Autodesk Inventor part; units mm, degrees
(part 3 of 3)
  spline S565 degree 2 poles (0.1635, 59.9365) (0.1635, 59.319) (1.0898, 58.6191) (1.9646, 58.6191) knots 0 0 0 1 2 2 2
  spline S566 degree 2 poles (1.9646, 58.6191) (2.8085, 58.6191) (3.6987, 59.1543) (3.6987, 59.7461) knots 0 0 0 1 2 2 2
  spline S567 degree 2 poles (3.6987, 59.7461) (3.6987, 60.06) (3.4106, 60.6981) (3.1687, 60.9811) knots 0 0 0 1 2 2 2
  line L445 (4.3265, 63.765) -> (4.3265, 62.9623)
  line L446 (4.3265, 62.9623) -> (-2.3065, 62.9623)
  line L447 (-2.3065, 62.9623) -> (-2.3065, 63.765)
  line L448 (-2.3065, 63.765) -> (4.3265, 63.765)
  spline S568 degree 2 poles (4.4346, 67.0121) (4.4346, 65.8697) (3.1533, 64.6141) (1.9697, 64.6141) knots 0 0 0 1 2 2 2
  spline S569 degree 2 poles (1.9697, 64.6141) (0.8068, 64.6141) (-0.5723, 65.8336) (-0.5723, 66.8165) knots 0 0 0 1 2 2 2
  spline S570 degree 2 poles (-0.5723, 66.8165) (-0.5723, 67.2591) (-0.315, 67.9435) (-0.0423, 68.1956) knots 0 0 0 1 2 2 2
  spline S571 degree 2 poles (-0.0423, 68.1956) (0.2304, 68.4529) (1.0177, 68.7256) (1.5889, 68.7256) knots 0 0 0 1 2 2 2
  line L449 (1.5889, 68.7256) -> (2.0263, 68.7256)
  line L450 (2.0263, 68.7256) -> (2.0263, 65.4271)
  spline S572 degree 2 poles (2.0263, 65.4271) (2.8548, 65.4271) (3.7348, 66.2608) (3.7348, 67.0018) knots 0 0 0 1 2 2 2
  spline S573 degree 2 poles (3.7348, 67.0018) (3.7348, 67.2642) (3.6164, 67.7736) (3.5238, 67.9795) knots 0 0 0 1 2 2 2
  spline S574 degree 2 poles (3.5238, 67.9795) (3.4209, 68.1956) (3.2408, 68.4941) (3.1584, 68.5918) knots 0 0 0 1 2 2 2
  line L451 (3.1584, 68.5918) -> (3.1584, 68.6381)
  line L452 (3.1584, 68.6381) -> (4.0332, 68.6381)
  spline S575 degree 2 poles (4.0332, 68.6381) (4.0898, 68.4992) (4.2545, 68.0772) (4.3008, 67.9126) knots 0 0 0 1 2 2 2
  spline S576 degree 2 poles (4.3008, 67.9126) (4.3677, 67.681) (4.4346, 67.3002) (4.4346, 67.0121) knots 0 0 0 1 2 2 2
  spline S577 degree 2 poles (1.414, 67.9435) (1.0898, 67.9332) (0.6164, 67.7994) (0.4568, 67.6707) knots 0 0 0 1 2 2 2
  spline S578 degree 2 poles (0.4568, 67.6707) (0.2767, 67.5318) (0.0863, 67.0944) (0.0863, 66.7702) knots 0 0 0 1 2 2 2
  spline S579 degree 2 poles (0.0863, 66.7702) (0.0863, 66.4512) (0.2767, 66.0035) (0.462, 65.8182) knots 0 0 0 1 2 2 2
  spline S580 degree 2 poles (0.462, 65.8182) (0.6524, 65.6381) (1.1104, 65.4529) (1.414, 65.4271) knots 0 0 0 1 2 2 2
  line L453 (1.414, 65.4271) -> (1.414, 67.9435)
  spline S581 degree 2 poles (10.3769, -6.4864) (10.7886, -6.4864) (11.5296, -6.7797) (11.7869, -7.0421) knots 0 0 0 1 2 2 2
  spline S582 degree 2 poles (11.7869, -7.0421) (12.1111, -7.3715) (12.4456, -8.2617) (12.4456, -8.9409) knots 0 0 0 1 2 2 2
  line L454 (12.4456, -8.9409) -> (12.4456, -9.6562)
  line L455 (12.4456, -9.6562) -> (14.8127, -9.6562)
  line L456 (14.8127, -9.6562) -> (14.8127, -10.5001)
  line L457 (14.8127, -10.5001) -> (8.4627, -10.5001)
  line L458 (8.4627, -10.5001) -> (8.4627, -8.9049)
  spline S583 degree 2 poles (8.4627, -8.9049) (8.4627, -8.3389) (8.6479, -7.5464) (8.8589, -7.2428) knots 0 0 0 1 2 2 2
  spline S584 degree 2 poles (8.8589, -7.2428) (9.1007, -6.8877) (9.8469, -6.4864) (10.3769, -6.4864) knots 0 0 0 1 2 2 2
  spline S585 degree 2 poles (10.4027, -7.3663) (10.0733, -7.3663) (9.5896, -7.5927) (9.4352, -7.8243) knots 0 0 0 1 2 2 2
  spline S586 degree 2 poles (9.4352, -7.8243) (9.3014, -8.025) (9.1934, -8.5601) (9.1934, -8.9564) knots 0 0 0 1 2 2 2
  line L459 (9.1934, -8.9564) -> (9.1934, -9.6562)
  line L460 (9.1934, -9.6562) -> (11.7251, -9.6562)
  line L461 (11.7251, -9.6562) -> (11.7251, -9.0799)
  spline S587 degree 2 poles (11.7251, -9.0799) (11.7251, -8.5653) (11.5605, -7.9324) (11.3443, -7.7265) knots 0 0 0 1 2 2 2
  spline S588 degree 2 poles (11.3443, -7.7265) (11.1539, -7.5361) (10.7063, -7.3663) (10.4027, -7.3663) knots 0 0 0 1 2 2 2
  line L462 (8.4627, -1.0781) -> (14.8127, -3.2651)
  line L463 (14.8127, -3.2651) -> (14.8127, -4.1759)
  line L464 (14.8127, -4.1759) -> (8.4627, -6.3629)
  line L465 (8.4627, -6.3629) -> (8.4627, -5.4572)
  line L466 (8.4627, -5.4572) -> (13.7372, -3.6973)
  line L467 (13.7372, -3.6973) -> (8.4627, -1.9374)
  line L468 (8.4627, -1.9374) -> (8.4627, -1.0781)
  spline S589 degree 2 poles (11.6377, 6.1004) (13.3461, 6.1004) (14.9465, 5.1073) (14.9465, 4.073) knots 0 0 0 1 2 2 2
  spline S590 degree 2 poles (14.9465, 4.073) (14.9465, 3.0232) (13.3152, 2.0403) (11.6428, 2.0403) knots 0 0 0 1 2 2 2
  spline S591 degree 2 poles (11.6428, 2.0403) (9.9241, 2.0403) (8.334, 3.0335) (8.334, 4.073) knots 0 0 0 1 2 2 2
  spline S592 degree 2 poles (8.334, 4.073) (8.334, 5.1176) (9.9807, 6.1004) (11.6377, 6.1004) knots 0 0 0 1 2 2 2
  spline S593 degree 2 poles (13.5725, 5.0095) (13.2586, 5.133) (12.2912, 5.2359) (11.6377, 5.2359) knots 0 0 0 1 2 2 2
  spline S594 degree 2 poles (11.6377, 5.2359) (10.9841, 5.2359) (10.0219, 5.133) (9.6977, 5.0044) knots 0 0 0 1 2 2 2
  spline S595 degree 2 poles (9.6977, 5.0044) (9.3735, 4.8757) (9.039, 4.428) (9.039, 4.073) knots 0 0 0 1 2 2 2
  spline S596 degree 2 poles (9.039, 4.073) (9.039, 3.7179) (9.3735, 3.2599) (9.708, 3.1261) knots 0 0 0 1 2 2 2
  spline S597 degree 2 poles (9.708, 3.1261) (10.0321, 2.9975) (11.0202, 2.9048) (11.6428, 2.9048) knots 0 0 0 1 2 2 2
  spline S598 degree 2 poles (11.6428, 2.9048) (12.3118, 2.9048) (13.2071, 2.9872) (13.5571, 3.121) knots 0 0 0 1 2 2 2
  spline S599 degree 2 poles (13.5571, 3.121) (13.8864, 3.2445) (14.2415, 3.7025) (14.2415, 4.073) knots 0 0 0 1 2 2 2
  spline S600 degree 2 poles (14.2415, 4.073) (14.2415, 4.4229) (13.907, 4.8809) (13.5725, 5.0095) knots 0 0 0 1 2 2 2
  line L469 (14.8127, 10.8295) -> (14.8127, 6.9135)
  line L470 (14.8127, 6.9135) -> (13.9121, 6.9135)
  spline S601 degree 2 poles (13.9121, 6.9135) (13.5159, 7.3354) (12.78, 8.0867) (12.3838, 8.4469) knots 0 0 0 1 2 2 2
  spline S602 degree 2 poles (12.3838, 8.4469) (11.5862, 9.1725) (10.6291, 9.7025) (10.1196, 9.7025) knots 0 0 0 1 2 2 2
  spline S603 degree 2 poles (10.1196, 9.7025) (9.852, 9.7025) (9.4507, 9.5379) (9.322, 9.3886) knots 0 0 0 1 2 2 2
  spline S604 degree 2 poles (9.322, 9.3886) (9.1934, 9.2394) (9.0647, 8.8483) (9.0647, 8.6116) knots 0 0 0 1 2 2 2
  spline S605 degree 2 poles (9.0647, 8.6116) (9.0647, 8.3852) (9.1779, 7.9221) (9.2654, 7.7111) knots 0 0 0 1 2 2 2
  spline S606 degree 2 poles (9.2654, 7.7111) (9.3375, 7.531) (9.5433, 7.1965) (9.6153, 7.0936) knots 0 0 0 1 2 2 2
  line L471 (9.6153, 7.0936) -> (9.6153, 7.0473)
  line L472 (9.6153, 7.0473) -> (8.7097, 7.0473)
  spline S607 degree 2 poles (8.7097, 7.0473) (8.581, 7.3097) (8.3289, 8.2514) (8.3289, 8.6734) knots 0 0 0 1 2 2 2
  spline S608 degree 2 poles (8.3289, 8.6734) (8.3289, 9.5636) (9.2706, 10.567) (10.0733, 10.567) knots 0 0 0 1 2 2 2
  spline S609 degree 2 poles (10.0733, 10.567) (10.449, 10.567) (11.0768, 10.3921) (11.3443, 10.2377) knots 0 0 0 1 2 2 2
  spline S610 degree 2 poles (11.3443, 10.2377) (11.6222, 10.0833) (12.1677, 9.6356) (12.4301, 9.3886) knots 0 0 0 1 2 2 2
  spline S611 degree 2 poles (12.4301, 9.3886) (12.8675, 8.9873) (13.8041, 8.0044) (14.0768, 7.7111) knots 0 0 0 1 2 2 2
  line L473 (14.0768, 7.7111) -> (14.0768, 10.8295)
  line L474 (14.0768, 10.8295) -> (14.8127, 10.8295)
  point P0 (0, 0)
  constraints: 2 end point, 2 midpoint, 1 vertical
extrude "Extrusion13" cut sketch "Sketch18" against normal blind 1.27
split "Split1" plane through (0, 0, 0) removes the side toward (-1, 0, 0)
sketch "Sketch24" plane through (19.05, -12.065, 27.94) normal (1, 0, 0) x (0, 0, -1)
  line L0 (-69.85, 100.965) -> (-57.15, 100.965) construction
  line L1 (-63.5, 100.965) -> (-63.5, 0) construction
  line L2 (-69.85, 0) -> (-40.2942, 0) construction
  line L3 (0, 20.955) -> (0, 0) construction
  line L4 (0, 6.0325) -> (-63.5, 6.0325) construction
  line L5 (0, 0) -> (-69.85, 0) construction
  point P0 (27.94, 12.065)
  point P1 (-63.5, 94.615)
  point P2 (-6.35, 6.0325)
  point P3 (-63.5, 69.215)
  point P4 (-63.5, 43.815)
  point P5 (-63.5, 18.415)
  point P6 (-31.75, 6.0325)
  point P7 (-57.15, 6.0325)
  dimension "d150" = 6.0325
  dimension "d151" = 6.35
  dimension "d152" = 6.35
  dimension "d155" = 25.4
  dimension "d162" = 25.4
  constraints: 5 point on line, 4 end point, 2 vertical, 1 horizontal, 1 midpoint, 1 perpendicular, 5 other
  measures "d150" distance between parallel lines of L4 L5
  measures "d151" distance from line of point (-63.5, 94.615) L0
  measures "d152" distance from line of point (-6.35, 6.033) L3
  measures "d155" distance of point (-63.5, 94.615) point (-63.5, 69.215)
  measures "d162" distance of point (-6.35, 6.033) point (-31.75, 6.033)
hole "Hole6" at (19.05, 82.55, 91.44) at (19.05, -6.0325, 34.29) at (19.05, 57.15, 91.44) at (19.05, 31.75, 91.44) at (19.05, 6.35, 91.44) at (19.05, -6.0325, 59.69) at (19.05, -6.0325, 85.09) direction (-1, 0, 0) diameter 5.1054 end through all clearance for "Hex Machine Screw" size "#10" standard "Ansi Unified Screw Threads"
equation "\"d0\" = innerWidth"
equation "\"d1\" = innerLength"
equation "\"d2\" = wallThickness"
equation "\"d3\" = wallThickness"
equation "\"d4\" = bottomThickness"
equation "\"d6\" = innerDepth"
equation "\"d8\" = holeCenterFromInnerWall"
equation "\"d9\" = holeCenterFromInnerWall"
equation "\"d104\" = armHeight"
equation "\"d120\" = hexSize"
equation "\"innerWidth\" = 43.18"
equation "\"innerLength\" = 107.95"
equation "\"innerDepth\" = 8.89"
equation "\"wallThickness\" = 6.35"
equation "\"postDiameter\" = 9.525"
equation "\"holeCenterFromInnerWall\" = 12.7"
equation "\"bottomThickness\" = 12.065"
equation "\"d17\" = postDiameter"
equation "\"exteriorWidth\" = innerWidth + 2 * wallThickness"
equation "\"exteriorLength\" = innerLength + 2 * wallThickness"
equation "\"exteriorHeight\" = innerDepth + bottomThickness"
equation "\"d24\" = postDiameter"
equation "\"lowerPostWidth\" = exteriorWidth"
equation "\"lowerPostLength\" = 50.8"
equation "\"lowerPostCenterX\" = 0.5 * exteriorLength"
equation "\"lowerPostHeight\" = 19.05"
equation "\"lowerPostCenterY\" = postDiameter"
equation "\"setScrewCenters\" = 0.333333 * exteriorWidth"
equation "\"printGap\" = 0.127"
equation "\"armHeight\" = 88.9"
equation "\"hexSize\" = 12.954"
body "Solid1"
